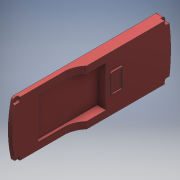
# Autodesk Inventor part: ET10
Saved by Autodesk Inventor 2016 (Build 200138000, 138)
## iProperties
Created: 2016-03-20
Part Number: ET10
Material: Genérico
Document SubType Name: Modeling
Designer: Usuario1
Density: 1 g/cm^3
Appearance: Valor por defecto
Author: Usuario1
Autodesk Inventor part; units mm, degrees
ref_plane "XZ Plane" through (0, 0, 0) normal (0, 1, 0) x (-1, 0, 0)
ref_plane "XY Plane" through (0, 0, 0) normal (0, 0, 1) x (1, 0, 0)
sketch "Boceto1" plane through (0, 0, 0) normal (1, 0, 0) x (0, 1, 0)
  line L0 (5.0799, -0.4268) -> (5.0799, -2.9809)
  line L1 (5.0799, -2.9809) -> (1.2627, -2.9809)
  line L2 (1.2627, -2.9809) -> (1.2627, -0.4268)
  line L3 (1.2627, -0.4268) -> (5.0799, -0.4268)
  line L4 (6.0017, -1.144) -> (6.0017, -2.2637)
  line L5 (6.0017, -2.2637) -> (5.4144, -2.2637)
  line L6 (5.4144, -2.2637) -> (5.4144, -1.144)
  line L7 (5.4144, -1.144) -> (6.0017, -1.144)
  arc A0 (-0.1462, -0.1163) -> (-0.1462, -3.2914) centre (6.7442, -1.7039) ccw
  arc A1 (-0.1462, -3.2914) -> (0, -3.4078) centre (0, -3.2578) ccw
  arc A2 (0, 0) -> (-0.1462, -0.1163) centre (0, -0.15) ccw
  arc A3 (9.0036, -3.2776) -> (9.0036, -0.1302) centre (-2.8031, -1.7039) ccw
  arc A4 (8.8549, -3.4078) -> (9.0036, -3.2776) centre (8.8549, -3.2578) ccw
  arc A5 (9.0036, -0.1302) -> (8.8549, 0) centre (8.8549, -0.15) ccw
  circle A6 centre (8.8549, -0.15) radius 0.092
  line L8 (8.7264, 0) -> (8.7264, -0.16)
  line L9 (9.0226, -0.28) -> (8.8464, -0.28)
  arc A7 (8.7264, -0.16) -> (8.8464, -0.28) centre (8.8464, -0.16) ccw
  circle A8 centre (0, -0.15) radius 0.092
  line L10 (0.1285, 0) -> (0.1285, -0.16)
  line L11 (-0.1818, -0.28) -> (0.0085, -0.28)
  arc A9 (0.0085, -0.28) -> (0.1285, -0.16) centre (0.0085, -0.16) ccw
  circle A10 centre (8.8549, -3.2578) radius 0.092
  line L12 (8.7264, -3.4078) -> (8.7264, -3.2478)
  line L13 (9.0226, -3.1278) -> (8.8464, -3.1278)
  arc A11 (8.8464, -3.1278) -> (8.7264, -3.2478) centre (8.8464, -3.2478) ccw
  circle A12 centre (0, -3.2578) radius 0.092
  line L14 (0.1285, -3.4078) -> (0.1285, -3.2478)
  line L15 (-0.1818, -3.1278) -> (0.0085, -3.1278)
  arc A13 (0.1285, -3.2478) -> (0.0085, -3.1278) centre (0.0085, -3.2478) ccw
  line L16 (8.8549, 0) -> (0, 0)
  line L17 (0, -3.4078) -> (8.8549, -3.4078)
  line L18 (5.8255, -1.144) -> (5.8255, -2.2637)
  line L19 (5.3143, -1.144) -> (5.3143, -2.2637)
  line L20 (5.358, -1.144) -> (5.358, -2.2637)
  line L21 (6.0582, -1.144) -> (6.0582, -2.2637)
  line L22 (6.1019, -1.144) -> (6.1019, -2.2637)
  line L23 (6.0017, -1.0439) -> (5.4144, -1.0439)
  line L24 (6.0017, -1.0876) -> (5.4144, -1.0876)
  line L25 (5.4219, -2.3636) -> (6.0017, -2.3639)
  line L26 (6.0017, -2.3201) -> (5.4144, -2.3201)
  arc A14 (6.0017, -2.3639) -> (6.1019, -2.2637) centre (6.0017, -2.2637) ccw
  arc A15 (6.0017, -2.3201) -> (6.0582, -2.2637) centre (6.0017, -2.2637) ccw
  arc A16 (6.0582, -1.144) -> (6.0017, -1.0876) centre (6.0017, -1.144) ccw
  arc A17 (6.1019, -1.144) -> (6.0017, -1.0439) centre (6.0017, -1.144) ccw
  arc A18 (5.4144, -1.0439) -> (5.3143, -1.144) centre (5.4144, -1.144) ccw
  arc A19 (5.4144, -1.0876) -> (5.358, -1.144) centre (5.4144, -1.144) ccw
  arc A20 (5.358, -2.2637) -> (5.4144, -2.3201) centre (5.4144, -2.2637) ccw
  arc A21 (5.3143, -2.2637) -> (5.4219, -2.3636) centre (5.4144, -2.2637) ccw
  line L27 (1.6627, -0.4268) -> (1.6627, -2.9809)
  line L28 (4.6799, -0.4268) -> (4.6799, -2.9809)
  line L29 (3.8847, -3.4078) -> (3.8847, -2.9809)
  line L30 (3.8847, -0.4268) -> (3.8847, 0)
  line L31 (2.98, -3.4078) -> (2.98, -2.9809)
  line L32 (2.98, -0.4268) -> (2.98, 0)
  line L33 (3.8847, -0.4268) -> (5.0799, -0.4268)
  line L34 (5.0799, -0.4268) -> (5.0799, -2.9809)
  line L35 (5.0799, -2.9809) -> (3.8847, -2.9809)
  constraints: 72 end point, 40 point on circle, 22 centre point, 20 point on line
extrude "Extrusión1" add sketch "Boceto1" along normal blind 0.15 contours L3 L30 L16 L8 A7 L9 A3 L13 A11 L12 L17 L29 L1 L0 | L4 L5 L18 L7 | L18 L5 L6 L7 | A18 L23 A17 L22 A14 L25 A21 L19 | A19 L24 A16 L21 A15 L26 A20 L20
ref_plane "Plano de trabajo1" through (-0.24, 0, 0) normal (1, 0, 0) x (0, 1, 0)
sketch "Boceto2" plane through (-0.24, 0, 0) normal (1, 0, 0) x (0, 1, 0)
  line L0 (5.0799, -0.4268) -> (5.0799, -2.9809)
  line L1 (5.0799, -2.9809) -> (1.2627, -2.9809)
  line L2 (1.2627, -2.9809) -> (1.2627, -0.4268)
  line L3 (1.2627, -0.4268) -> (5.0799, -0.4268)
  line L4 (6.0017, -1.144) -> (6.0017, -2.2637)
  line L5 (6.0017, -2.2637) -> (5.4144, -2.2637)
  line L6 (5.4144, -2.2637) -> (5.4144, -1.144)
  line L7 (5.4144, -1.144) -> (6.0017, -1.144)
  arc A0 (-0.1462, -0.1163) -> (-0.1462, -3.2914) centre (6.7442, -1.7039) ccw
  arc A1 (-0.1462, -3.2914) -> (0, -3.4078) centre (0, -3.2578) ccw
  arc A2 (0, 0) -> (-0.1462, -0.1163) centre (0, -0.15) ccw
  arc A3 (9.0036, -3.2776) -> (9.0036, -0.1302) centre (-2.8031, -1.7039) ccw
  arc A4 (8.8549, -3.4078) -> (9.0036, -3.2776) centre (8.8549, -3.2578) ccw
  arc A5 (9.0036, -0.1302) -> (8.8549, 0) centre (8.8549, -0.15) ccw
  circle A6 centre (8.8549, -0.15) radius 0.092
  line L8 (8.7264, 0) -> (8.7264, -0.16)
  line L9 (9.0226, -0.28) -> (8.8464, -0.28)
  arc A7 (8.7264, -0.16) -> (8.8464, -0.28) centre (8.8464, -0.16) ccw
  circle A8 centre (0, -0.15) radius 0.092
  line L10 (0.1285, 0) -> (0.1285, -0.16)
  line L11 (-0.1818, -0.28) -> (0.0085, -0.28)
  arc A9 (0.0085, -0.28) -> (0.1285, -0.16) centre (0.0085, -0.16) ccw
  circle A10 centre (8.8549, -3.2578) radius 0.092
  line L12 (8.7264, -3.4078) -> (8.7264, -3.2478)
  line L13 (9.0226, -3.1278) -> (8.8464, -3.1278)
  arc A11 (8.8464, -3.1278) -> (8.7264, -3.2478) centre (8.8464, -3.2478) ccw
  circle A12 centre (0, -3.2578) radius 0.092
  line L14 (0.1285, -3.4078) -> (0.1285, -3.2478)
  line L15 (-0.1818, -3.1278) -> (0.0085, -3.1278)
  arc A13 (0.1285, -3.2478) -> (0.0085, -3.1278) centre (0.0085, -3.2478) ccw
  line L16 (8.8549, 0) -> (0, 0)
  line L17 (0, -3.4078) -> (8.8549, -3.4078)
  line L18 (5.8255, -1.144) -> (5.8255, -2.2637)
  line L19 (5.3143, -1.144) -> (5.3143, -2.2637)
  line L20 (5.358, -1.144) -> (5.358, -2.2637)
  line L21 (6.0582, -1.144) -> (6.0582, -2.2637)
  line L22 (6.1019, -1.144) -> (6.1019, -2.2637)
  line L23 (6.0017, -1.0439) -> (5.4144, -1.0439)
  line L24 (6.0017, -1.0876) -> (5.4144, -1.0876)
  line L25 (5.4219, -2.3636) -> (6.0017, -2.3639)
  line L26 (6.0017, -2.3201) -> (5.4144, -2.3201)
  arc A14 (6.0017, -2.3639) -> (6.1019, -2.2637) centre (6.0017, -2.2637) ccw
  arc A15 (6.0017, -2.3201) -> (6.0582, -2.2637) centre (6.0017, -2.2637) ccw
  arc A16 (6.0582, -1.144) -> (6.0017, -1.0876) centre (6.0017, -1.144) ccw
  arc A17 (6.1019, -1.144) -> (6.0017, -1.0439) centre (6.0017, -1.144) ccw
  arc A18 (5.4144, -1.0439) -> (5.3143, -1.144) centre (5.4144, -1.144) ccw
  arc A19 (5.4144, -1.0876) -> (5.358, -1.144) centre (5.4144, -1.144) ccw
  arc A20 (5.358, -2.2637) -> (5.4144, -2.3201) centre (5.4144, -2.2637) ccw
  arc A21 (5.3143, -2.2637) -> (5.4219, -2.3636) centre (5.4144, -2.2637) ccw
  line L27 (1.6627, -0.4268) -> (1.6627, -2.9809)
  line L28 (4.6799, -0.4268) -> (4.6799, -2.9809)
  line L29 (3.8847, -3.4078) -> (3.8847, -2.9809)
  line L30 (3.8847, -0.4268) -> (3.8847, 0)
  line L31 (2.98, -3.4078) -> (2.98, -2.9809)
  line L32 (2.98, -0.4268) -> (2.98, 0)
  line L33 (3.8847, -0.4268) -> (5.0799, -0.4268)
  line L34 (5.0799, -0.4268) -> (5.0799, -2.9809)
  line L35 (5.0799, -2.9809) -> (3.8847, -2.9809)
  line L36 (5.0799, -0.4268) -> (5.0799, -2.9809) projected
  line L37 (3.8847, -0.4268) -> (5.0799, -0.4268) projected
  line L38 (3.8847, 0) -> (3.8847, -0.4268) projected
  line L39 (8.7264, 0) -> (3.8847, 0) projected
  line L40 (8.7264, -0.16) -> (8.7264, 0) projected
  arc A22 (8.7264, -0.16) -> (8.8464, -0.28) centre (8.8464, -0.16) ccw projected
  line L41 (9.0226, -0.28) -> (8.8464, -0.28) projected
  arc A23 (9.0226, -3.1278) -> (9.0226, -0.28) centre (-2.8031, -1.7039) ccw projected
  line L42 (8.8464, -3.1278) -> (9.0226, -3.1278) projected
  arc A24 (8.8464, -3.1278) -> (8.7264, -3.2478) centre (8.8464, -3.2478) ccw projected
  line L43 (8.7264, -3.4078) -> (8.7264, -3.2478) projected
  line L44 (3.8847, -3.4078) -> (8.7264, -3.4078) projected
  line L45 (3.8847, -2.9809) -> (3.8847, -3.4078) projected
  line L46 (5.0799, -2.9809) -> (3.8847, -2.9809) projected
  line L47 (0, -3.4078) -> (2.98, -3.4078)
  line L48 (2.98, 0) -> (0, 0)
  line L49 (2.98, -0.4268) -> (2.98, -2.9809)
  point P0 (0, 0)
  constraints: 78 end point, 40 point on circle, 22 centre point, 20 point on line, 3 collinear
extrude "Extrusión2" add sketch "Boceto2" against normal blind 0.15 contours L49 L1 L27 L3 | L3 L2 L1 L31 L17 L14 A13 L15 A0 L11 A9 L10 L16 L32 | L27 L1 L2 L3 | L17 A1 A0 L15 A13 L14 | A12
sketch "Boceto3" plane through (-0.24, 0.1285, 0) normal (0, 0, 1) x (1, 0, 0)
  line L0 (0.24, 8.5978) -> (0.24, 3.7561) projected
  line L1 (0.24, 3.7561) -> (0.39, 3.7561) projected
  line L2 (0.39, 8.5978) -> (0.39, 3.7561) projected
  line L3 (0.24, 8.5978) -> (0.39, 8.5978) projected
  line L4 (0, 2.8515) -> (0, 0) projected
  line L5 (0, 2.8515) -> (-0.15, 2.8515) projected
  line L6 (-0.15, 0) -> (-0.15, 2.8515) projected
  line L7 (0, 0) -> (-0.15, 0) projected
  arc A0 (0.24, 3.7561) -> (-0.15, 2.8515) centre (1.386, 2.7257) ccw
  line L8 (0.24, 3.7561) -> (0.39, 3.7561) projected
  line L9 (0.24, 3.7561) -> (0.39, 3.7561)
  line L10 (-0.15, 0) -> (-0.15, 2.8515) projected
  line L11 (0, 2.8515) -> (0, 0) projected
  line L12 (-0.15, 2.8515) -> (0, 2.8515)
  arc A1 (0.39, 3.7561) -> (0, 2.8515) centre (1.536, 2.7257) ccw
  line L13 (0.24, 3.7561) -> (0.39, 3.7561)
  line L14 (-0.15, 2.8515) -> (0, 2.8515)
  point P0 (0.24, -0.1285)
  constraints: 8 end point, 6 point on circle, 2 centre point, 2 equal length, 2 horizontal, 2 point on line
extrude "Extrusión3" add sketch "Boceto3" against normal blind 3.4078 contours L1 A1 L5 A0
sketch "Boceto4" plane through (0.15, 0, 0) normal (1, 0, 0) x (0, 0, -1)
  line L0 (0.4268, 5.0799) -> (2.9809, 5.0799) projected
  line L1 (2.9809, 5.0799) -> (2.9809, 3.8847) projected
  line L2 (2.9809, 3.8847) -> (3.4078, 3.8847) projected
  line L3 (3.4078, 3.8847) -> (3.4078, 8.7264) projected
  line L4 (3.4078, 8.7264) -> (3.2478, 8.7264) projected
  arc A0 (3.1278, 8.8464) -> (3.2478, 8.7264) centre (3.2478, 8.8464) ccw projected
  line L5 (3.1278, 8.8464) -> (3.1278, 9.0226) projected
  arc A1 (3.1278, 9.0226) -> (0.28, 9.0226) centre (1.7039, -2.8031) ccw projected
  line L6 (0.28, 9.0226) -> (0.28, 8.8464) projected
  arc A2 (0.16, 8.7264) -> (0.28, 8.8464) centre (0.16, 8.8464) ccw projected
  line L7 (0.16, 8.7264) -> (0, 8.7264) projected
  line L8 (0, 8.7264) -> (0, 3.8847) projected
  line L9 (0, 3.8847) -> (0.4268, 3.8847) projected
  line L10 (0.4268, 3.8847) -> (0.4268, 5.0799) projected
  line L11 (0.4268, 5.0799) -> (2.9809, 5.0799)
  line L12 (2.9809, 5.0799) -> (2.9809, 1.2627)
  line L13 (2.9809, 1.2627) -> (0.4268, 1.2627)
  line L14 (0.4268, 1.2627) -> (0.4268, 5.0799)
  line L15 (1.144, 6.0017) -> (2.2637, 6.0017)
  line L16 (2.2637, 6.0017) -> (2.2637, 5.4144)
  line L17 (2.2637, 5.4144) -> (1.144, 5.4144)
  line L18 (1.144, 5.4144) -> (1.144, 6.0017)
  arc A3 (0.1163, -0.1462) -> (3.2914, -0.1462) centre (1.7039, 6.7442) ccw
  arc A4 (3.2914, -0.1462) -> (3.4078, 0) centre (3.2578, 0) ccw
  arc A5 (0, 0) -> (0.1163, -0.1462) centre (0.15, 0) ccw
  arc A6 (3.2776, 9.0036) -> (0.1302, 9.0036) centre (1.7039, -2.8031) ccw
  arc A7 (3.4078, 8.8549) -> (3.2776, 9.0036) centre (3.2578, 8.8549) ccw
  arc A8 (0.1302, 9.0036) -> (0, 8.8549) centre (0.15, 8.8549) ccw
  circle A9 centre (0.15, 8.8549) radius 0.092
  line L19 (0, 8.7264) -> (0.16, 8.7264)
  line L20 (0.28, 9.0226) -> (0.28, 8.8464)
  arc A10 (0.16, 8.7264) -> (0.28, 8.8464) centre (0.16, 8.8464) ccw
  circle A11 centre (0.15, 0) radius 0.092
  line L21 (0, 0.1285) -> (0.16, 0.1285)
  line L22 (0.28, -0.1818) -> (0.28, 0.0085)
  arc A12 (0.28, 0.0085) -> (0.16, 0.1285) centre (0.16, 0.0085) ccw
  circle A13 centre (3.2578, 8.8549) radius 0.092
  line L23 (3.4078, 8.7264) -> (3.2478, 8.7264)
  line L24 (3.1278, 9.0226) -> (3.1278, 8.8464)
  arc A14 (3.1278, 8.8464) -> (3.2478, 8.7264) centre (3.2478, 8.8464) ccw
  circle A15 centre (3.2578, 0) radius 0.092
  line L25 (3.4078, 0.1285) -> (3.2478, 0.1285)
  line L26 (3.1278, -0.1818) -> (3.1278, 0.0085)
  arc A16 (3.2478, 0.1285) -> (3.1278, 0.0085) centre (3.2478, 0.0085) ccw
  line L27 (0, 8.8549) -> (0, 0)
  line L28 (3.4078, 0) -> (3.4078, 8.8549)
  line L29 (1.144, 5.8255) -> (2.2637, 5.8255)
  line L30 (1.144, 5.3143) -> (2.2637, 5.3143)
  line L31 (1.144, 5.358) -> (2.2637, 5.358)
  line L32 (1.144, 6.0582) -> (2.2637, 6.0582)
  line L33 (1.144, 6.1019) -> (2.2637, 6.1019)
  line L34 (1.0439, 6.0017) -> (1.0439, 5.4144)
  line L35 (1.0876, 6.0017) -> (1.0876, 5.4144)
  line L36 (2.3636, 5.4219) -> (2.3639, 6.0017)
  line L37 (2.3201, 6.0017) -> (2.3201, 5.4144)
  arc A17 (2.3639, 6.0017) -> (2.2637, 6.1019) centre (2.2637, 6.0017) ccw
  arc A18 (2.3201, 6.0017) -> (2.2637, 6.0582) centre (2.2637, 6.0017) ccw
  arc A19 (1.144, 6.0582) -> (1.0876, 6.0017) centre (1.144, 6.0017) ccw
  arc A20 (1.144, 6.1019) -> (1.0439, 6.0017) centre (1.144, 6.0017) ccw
  arc A21 (1.0439, 5.4144) -> (1.144, 5.3143) centre (1.144, 5.4144) ccw
  arc A22 (1.0876, 5.4144) -> (1.144, 5.358) centre (1.144, 5.4144) ccw
  arc A23 (2.2637, 5.358) -> (2.3201, 5.4144) centre (2.2637, 5.4144) ccw
  arc A24 (2.2637, 5.3143) -> (2.3636, 5.4219) centre (2.2637, 5.4144) ccw
  line L38 (0.4268, 1.6627) -> (2.9809, 1.6627)
  line L39 (0.4268, 4.6799) -> (2.9809, 4.6799)
  line L40 (3.4078, 3.8847) -> (2.9809, 3.8847)
  line L41 (0.4268, 3.8847) -> (0, 3.8847)
  line L42 (3.4078, 2.98) -> (2.9809, 2.98)
  line L43 (0.4268, 2.98) -> (0, 2.98)
  line L44 (0.4268, 3.8847) -> (0.4268, 5.0799)
  line L45 (0.4268, 5.0799) -> (2.9809, 5.0799)
  line L46 (2.9809, 5.0799) -> (2.9809, 3.8847)
  point P0 (0, 0)
  constraints: 72 end point, 40 point on circle, 22 centre point, 20 point on line
extrude "Extrusión4" cut sketch "Boceto4" against normal blind 3.4078 contours L39 L1 L12 L38 L14 L10 | L38 L12 L13 L14
ref_plane "Plano de trabajo2" through (-0.52, 0, 0) normal (1, 0, 0) x (0, 1, 0)
sketch "Boceto5" plane through (-0.52, 0, 0) normal (1, 0, 0) x (0, 1, 0)
  arc A0 (9.0226, -3.1278) -> (9.0226, -0.28) centre (-2.8031, -1.7039) ccw projected
  line L0 (5.0799, -0.4268) -> (5.0799, -2.9809)
  line L1 (5.0799, -2.9809) -> (1.2627, -2.9809)
  line L2 (1.2627, -2.9809) -> (1.2627, -0.4268)
  line L3 (1.2627, -0.4268) -> (5.0799, -0.4268)
  line L4 (6.0017, -1.144) -> (6.0017, -2.2637)
  line L5 (6.0017, -2.2637) -> (5.4144, -2.2637)
  line L6 (5.4144, -2.2637) -> (5.4144, -1.144)
  line L7 (5.4144, -1.144) -> (6.0017, -1.144)
  arc A1 (-0.1462, -0.1163) -> (-0.1462, -3.2914) centre (6.7442, -1.7039) ccw
  arc A2 (-0.1462, -3.2914) -> (0, -3.4078) centre (0, -3.2578) ccw
  arc A3 (0, 0) -> (-0.1462, -0.1163) centre (0, -0.15) ccw
  arc A4 (9.0036, -3.2776) -> (9.0036, -0.1302) centre (-2.8031, -1.7039) ccw
  arc A5 (8.8549, -3.4078) -> (9.0036, -3.2776) centre (8.8549, -3.2578) ccw
  arc A6 (9.0036, -0.1302) -> (8.8549, 0) centre (8.8549, -0.15) ccw
  circle A7 centre (8.8549, -0.15) radius 0.092
  line L8 (8.7264, 0) -> (8.7264, -0.16)
  line L9 (9.0226, -0.28) -> (8.8464, -0.28)
  arc A8 (8.7264, -0.16) -> (8.8464, -0.28) centre (8.8464, -0.16) ccw
  circle A9 centre (0, -0.15) radius 0.092
  line L10 (0.1285, 0) -> (0.1285, -0.16)
  line L11 (-0.1818, -0.28) -> (0.0085, -0.28)
  arc A10 (0.0085, -0.28) -> (0.1285, -0.16) centre (0.0085, -0.16) ccw
  circle A11 centre (8.8549, -3.2578) radius 0.092
  line L12 (8.7264, -3.4078) -> (8.7264, -3.2478)
  line L13 (9.0226, -3.1278) -> (8.8464, -3.1278)
  arc A12 (8.8464, -3.1278) -> (8.7264, -3.2478) centre (8.8464, -3.2478) ccw
  circle A13 centre (0, -3.2578) radius 0.092
  line L14 (0.1285, -3.4078) -> (0.1285, -3.2478)
  line L15 (-0.1818, -3.1278) -> (0.0085, -3.1278)
  arc A14 (0.1285, -3.2478) -> (0.0085, -3.1278) centre (0.0085, -3.2478) ccw
  line L16 (8.8549, 0) -> (0, 0)
  line L17 (0, -3.4078) -> (8.8549, -3.4078)
  line L18 (5.8255, -1.144) -> (5.8255, -2.2637)
  line L19 (5.3143, -1.144) -> (5.3143, -2.2637)
  line L20 (5.358, -1.144) -> (5.358, -2.2637)
  line L21 (6.0582, -1.144) -> (6.0582, -2.2637)
  line L22 (6.1019, -1.144) -> (6.1019, -2.2637)
  line L23 (6.0017, -1.0439) -> (5.4144, -1.0439)
  line L24 (6.0017, -1.0876) -> (5.4144, -1.0876)
  line L25 (5.4219, -2.3636) -> (6.0017, -2.3639)
  line L26 (6.0017, -2.3201) -> (5.4144, -2.3201)
  arc A15 (6.0017, -2.3639) -> (6.1019, -2.2637) centre (6.0017, -2.2637) ccw
  arc A16 (6.0017, -2.3201) -> (6.0582, -2.2637) centre (6.0017, -2.2637) ccw
  arc A17 (6.0582, -1.144) -> (6.0017, -1.0876) centre (6.0017, -1.144) ccw
  arc A18 (6.1019, -1.144) -> (6.0017, -1.0439) centre (6.0017, -1.144) ccw
  arc A19 (5.4144, -1.0439) -> (5.3143, -1.144) centre (5.4144, -1.144) ccw
  arc A20 (5.4144, -1.0876) -> (5.358, -1.144) centre (5.4144, -1.144) ccw
  arc A21 (5.358, -2.2637) -> (5.4144, -2.3201) centre (5.4144, -2.2637) ccw
  arc A22 (5.3143, -2.2637) -> (5.4219, -2.3636) centre (5.4144, -2.2637) ccw
  line L27 (1.6627, -0.4268) -> (1.6627, -2.9809)
  line L28 (4.6799, -0.4268) -> (4.6799, -2.9809)
  line L29 (3.8847, -3.4078) -> (3.8847, -2.9809)
  line L30 (3.8847, -0.4268) -> (3.8847, 0)
  line L31 (2.98, -3.4078) -> (2.98, -2.9809)
  line L32 (2.98, -0.4268) -> (2.98, 0)
  line L33 (3.8847, -0.4268) -> (5.0799, -0.4268)
  line L34 (5.0799, -0.4268) -> (5.0799, -2.9809)
  line L35 (5.0799, -2.9809) -> (3.8847, -2.9809)
  arc A23 (0, -0.15) -> (0, -3.2578) centre (6.7442, -1.7039) ccw
  line L36 (0, -3.2578) -> (8.8549, -3.2578)
  arc A24 (8.8549, -3.2578) -> (8.8549, -0.15) centre (-2.8031, -1.7039) ccw
  line L37 (8.8549, -0.15) -> (0, -0.15)
  line L38 (2.98, 0) -> (0.1285, 0) projected
  line L39 (0.1285, 0) -> (8.7264, 0)
  line L40 (8.7264, 0) -> (8.7264, -0.15)
  line L41 (8.7264, -0.15) -> (0.1285, -0.15)
  line L42 (0.1285, -0.15) -> (0.1285, 0)
  line L43 (8.7264, -3.4078) -> (0.1285, -3.4078)
  line L44 (0.1285, -3.4078) -> (0.1285, -3.2578)
  line L45 (0.1285, -3.2578) -> (8.7264, -3.2578)
  line L46 (8.7264, -3.2578) -> (8.7264, -3.4078)
  line L47 (-0.0286, -3.1278) -> (-0.1818, -3.1278)
  arc A25 (-0.1818, -0.28) -> (-0.1462, -3.2914) centre (6.7442, -1.7039) ccw projected
  line L48 (-0.0286, -0.28) -> (-0.1818, -0.28)
  line L49 (9.0226, -0.28) -> (8.8715, -0.28)
  line L50 (9.0226, -0.28) -> (8.8464, -0.28) projected
  line L51 (9.0226, -3.1278) -> (8.8715, -3.1278)
  line L52 (8.8464, -3.1278) -> (9.0226, -3.1278) projected
  arc A26 (0, 0) -> (-0.1462, -0.1163) centre (0, -0.15) ccw
  line L53 (0.0085, -0.28) -> (-0.0286, -0.28)
  line L54 (-0.0286, -0.28) -> (-0.1818, -0.28)
  line L55 (0.1285, -0.16) -> (0.1285, -0.15)
  arc A27 (0.0085, -0.28) -> (0.1285, -0.16) centre (0.0085, -0.16) ccw
  arc A28 (-0.1462, -0.1163) -> (-0.1818, -0.28) centre (6.7442, -1.7039) ccw
  point P0 (0, 0)
  dimension "d10" = 0.15
  constraints: 106 end point, 54 point on circle, 28 point on line, 27 centre point, 4 horizontal, 4 parallel, 3 collinear, 2 perpendicular, 1 concentric, 3 other
  measures "d10" distance between parallel lines of L16 L37
extrude "Extrusión5" add sketch "Boceto5" along normal blind 0.13 contours L13 A24 L9 A0 | A4 A5 L17 L12 L36 A11 A24 L13 | L9 A24 A7 L37 L8 L16 A6 A4 | A24 A11 L36 L12 A12 L13 | L9 A8 L8 L37 A7 A24 | A24 L36 A11 | A11 L36 A24 | A24 L37 A7 | A7 L37 A24 | L17 L29 L36 L12 | L8 L37 L30 L16 | L17 L31 L36 L29 | L30 L37 L32 L16 | L17 L14 L36 L31 | L32 L37 L10 L16 | L17 A2 A1 L15 A23 A13 L36 L14 | L10 L37 A9 A23 L11 A1 A3 L16 | L36 A13 A23 L15 A14 L14 | L10 A10 L11 A23 A9 L37 | L36 A23 A13 | A13 A23 L36 | L37 A23 A9 | A9 A23 L37 | A1 L11 A23 L15
sketch "Boceto6" plane through (-0.39, 0, 0) normal (1, 0, 0) x (0, 0, -1)
  line L0 (0, 2.98) -> (0.15, 2.98) projected
  line L1 (0.15, 2.98) -> (0.15, 8.7264) projected
  line L2 (0.15, 8.7264) -> (0.16, 8.7264) projected
  arc A0 (0.16, 8.7264) -> (0.28, 8.8464) centre (0.16, 8.8464) ccw projected
  line L3 (0.28, 8.8464) -> (0.28, 8.8715) projected
  arc A1 (3.1278, 8.8715) -> (0.28, 8.8715) centre (1.7039, -2.8031) ccw projected
  line L4 (3.1278, 8.8715) -> (3.1278, 8.8464) projected
  arc A2 (3.1278, 8.8464) -> (3.2478, 8.7264) centre (3.2478, 8.8464) ccw projected
  line L5 (3.2478, 8.7264) -> (3.2578, 8.7264) projected
  line L6 (3.2578, 8.7264) -> (3.2578, 2.98) projected
  line L7 (3.2578, 2.98) -> (3.4078, 2.98) projected
  line L8 (3.4078, 2.98) -> (3.4078, 8.7264) projected
  line L9 (3.4078, 8.7264) -> (3.4078, 8.8549) projected
  arc A3 (3.4078, 8.8549) -> (3.2776, 9.0036) centre (3.2578, 8.8549) ccw projected
  arc A4 (3.2776, 9.0036) -> (0.1302, 9.0036) centre (1.7039, -2.8031) ccw projected
  arc A5 (0.1302, 9.0036) -> (0, 8.8549) centre (0.15, 8.8549) ccw projected
  line L10 (0, 8.8549) -> (0, 2.98) projected
  point P0 (0, 0)
extrude "Extrusión6" add sketch "Boceto6" along normal blind 0.15
sketch "Boceto7" plane through (-0.24, 0, 0) normal (1, 0, 0) x (0, 0, -1)
  line L0 (3.4078, 3.5281) -> (3.2578, 3.5281) projected
  line L1 (3.4078, 3.5281) -> (3.4078, 8.7264) projected
  line L2 (3.4078, 8.7264) -> (3.4078, 8.8549) projected
  arc A0 (3.4078, 8.8549) -> (3.2776, 9.0036) centre (3.2578, 8.8549) ccw projected
  arc A1 (3.2776, 9.0036) -> (0.1302, 9.0036) centre (1.7039, -2.8031) ccw projected
  arc A2 (0.1302, 9.0036) -> (0, 8.8549) centre (0.15, 8.8549) ccw projected
  line L3 (0, 8.8549) -> (0, 3.5281) projected
  line L4 (0.15, 3.5281) -> (0, 3.5281) projected
  line L5 (0.15, 3.5281) -> (0.15, 8.7264) projected
  line L6 (0.15, 8.7264) -> (0.16, 8.7264) projected
  arc A3 (0.16, 8.7264) -> (0.28, 8.8464) centre (0.16, 8.8464) ccw projected
  line L7 (0.28, 8.8464) -> (0.28, 8.8715) projected
  arc A4 (3.1278, 8.8715) -> (0.28, 8.8715) centre (1.7039, -2.8031) ccw projected
  line L8 (3.1278, 8.8715) -> (3.1278, 8.8464) projected
  arc A5 (3.1278, 8.8464) -> (3.2478, 8.7264) centre (3.2478, 8.8464) ccw projected
  line L9 (3.2478, 8.7264) -> (3.2578, 8.7264) projected
  line L10 (3.2578, 8.7264) -> (3.2578, 3.5281) projected
  point P0 (0, 0)
extrude "Extrusión7" add sketch "Boceto7" along normal blind 0.15
sketch "Boceto8" plane through (-0.09, 0, 0) normal (1, 0, 0) x (0, 0, -1)
  line L0 (0.15, 3.7748) -> (0, 3.7748) projected
  line L1 (0.15, 3.7748) -> (0.15, 8.7264) projected
  line L2 (0.15, 8.7264) -> (0.16, 8.7264) projected
  arc A0 (0.16, 8.7264) -> (0.28, 8.8464) centre (0.16, 8.8464) ccw projected
  line L3 (0.28, 8.8464) -> (0.28, 8.8715) projected
  arc A1 (3.1278, 8.8715) -> (0.28, 8.8715) centre (1.7039, -2.8031) ccw projected
  line L4 (3.1278, 8.8715) -> (3.1278, 8.8464) projected
  arc A2 (3.1278, 8.8464) -> (3.2478, 8.7264) centre (3.2478, 8.8464) ccw projected
  line L5 (3.2478, 8.7264) -> (3.2578, 8.7264) projected
  line L6 (3.2578, 8.7264) -> (3.2578, 3.7748) projected
  line L7 (3.4078, 3.7748) -> (3.2578, 3.7748) projected
  line L8 (3.4078, 3.7748) -> (3.4078, 8.7264) projected
  line L9 (3.4078, 8.7264) -> (3.4078, 8.8549) projected
  arc A3 (3.4078, 8.8549) -> (3.2776, 9.0036) centre (3.2578, 8.8549) ccw projected
  arc A4 (3.2776, 9.0036) -> (0.1302, 9.0036) centre (1.7039, -2.8031) ccw projected
  arc A5 (0.1302, 9.0036) -> (0, 8.8549) centre (0.15, 8.8549) ccw projected
  line L10 (0, 8.8549) -> (0, 3.7748) projected
  point P0 (0, 0)
extrude "Extrusión8" add sketch "Boceto8" along normal blind 0.15
sketch "Boceto9" plane through (0.15, 5.0799, -0.4268) normal (0, 0, -1) x (-1, 0, 0)
  line L0 (0.15, -1.1953) -> (0.15, 0) projected
  line L1 (0.15, 0) -> (0.15, 0.15)
  line L2 (0.54, -2.0999) -> (0.54, -3.8173) projected
  line L3 (0.54, -3.8173) -> (0.54, -3.9673)
  line L4 (0.54, -3.9673) -> (0.67, -3.9673)
  line L5 (0.67, -4.9514) -> (0.67, 3.6464) projected
  line L6 (0.15, 0.15) -> (0.67, 0.15)
  line L7 (0.67, 0.15) -> (0.67, -3.9673)
  arc A0 (0.54, -2.0999) -> (0.15, -1.1953) centre (-0.996, -2.2257) ccw projected
  point P0 (0.15, -5.0799)
  dimension "d19" = 0.15
  dimension "d20" = 0.15
  dimension "d21" = 0.13
  constraints: 10 end point, 2 point on line, 2 vertical, 1 collinear, 1 horizontal
  measures "d19" distance of L0.end L1.end
  measures "d20" distance of L2.end L3.end
  measures "d21" distance of L3.end L4.end
extrude "Extrusión9" add sketch "Boceto9" against normal blind 0.15
sketch "Boceto10" plane through (0, 5.0799, -2.9809) normal (0, 0, 1) x (1, 0, 0)
  line L0 (0, 0) -> (0.15, 0) projected
  line L1 (0.15, -1.1953) -> (0.15, 0) projected
  arc A0 (0.15, -1.1953) -> (-0.24, -2.0999) centre (1.296, -2.2257) ccw projected
  line L2 (-0.24, -3.8173) -> (-0.24, -2.0999) projected
  line L3 (-0.24, -3.8173) -> (-0.39, -3.8173) projected
  line L4 (-0.39, -3.9673) -> (-0.39, -3.8173) projected
  line L5 (-0.39, -3.9673) -> (-0.52, -3.9673) projected
  line L6 (-0.52, -3.9673) -> (-0.52, 0.15) projected
  line L7 (-0.52, 0.15) -> (0, 0.15) projected
  line L8 (0, 0) -> (0, 0.15) projected
  point P0 (0, -5.0799)
extrude "Extrusión10" add sketch "Boceto10" against normal blind 0.15
sketch "Boceto11" plane through (0.15, 5.0799, -0.4268) normal (0, 0, -1) x (-1, 0, 0)
  line L0 (0.67, 0.15) -> (0.67, -3.9673) projected
  line L1 (0.15, 0.15) -> (0.67, 0.15) projected
  arc A0 (0.54, -2.0999) -> (0.15, -1.1953) centre (-0.996, -2.2257) ccw projected
  line L2 (0.15, 0.15) -> (0.15, -1.1953) projected
  line L3 (0.15, 0.15) -> (0.67, 0.15) projected
  line L4 (0.67, 0.15) -> (0.67, -3.9673) projected
  line L5 (0.67, -3.9673) -> (0.54, -3.9673) projected
  line L6 (0.54, -2.0999) -> (0.54, -3.9673) projected
  line L7 (0.54, -2.0999) -> (0.54, -3.9673) projected
  line L8 (0.54, -3.9673) -> (0.67, -3.9673)
  line L9 (0.67, -3.9673) -> (0.67, 0.15)
  line L10 (0.67, 0.15) -> (0.54, 0.15)
  line L11 (0.54, 0.15) -> (0.54, -3.9673)
  point P0 (0.15, -5.0799)
  constraints: 8 end point, 2 parallel, 1 horizontal, 1 perpendicular
extrude "Extrusión11" add sketch "Boceto11" along normal blind 2.6 contours L0 L5 L6 L11 L1
sketch "Boceto12" plane through (-0.52, 5.2299, -0.2768) normal (0, 1, 0) x (1, 0, 0)
  line L0 (0, 0) -> (0, 2.8541) projected
  line L1 (0.52, 0) -> (0, 0) projected
  line L2 (0.52, 0.15) -> (0.52, 0) projected
  line L3 (0.13, 0.15) -> (0.52, 0.15) projected
  line L4 (0.13, 0.15) -> (0.13, 2.7041) projected
  line L5 (0.13, 2.7041) -> (0.52, 2.7041) projected
  line L6 (0.52, 2.8541) -> (0.52, 2.7041) projected
  line L7 (0, 2.8541) -> (0.52, 2.8541) projected
  line L8 (0.52, 0.15) -> (0.52, 2.7041) projected
  line L9 (0.52, 2.8541) -> (0.52, 2.7041) projected
  line L10 (0.52, 0.15) -> (0.52, 2.7041)
  line L11 (0.52, 0.15) -> (0.13, 0.15)
  line L12 (0.13, 0.15) -> (0.13, 2.7041)
  line L13 (0.13, 2.7041) -> (0.52, 2.7041)
  line L14 (0.52, 2.7041) -> (0.52, 0.15)
  point P0 (0.52, -0.2768)
  constraints: 10 end point, 2 parallel, 1 horizontal, 1 perpendicular, 1 vertical
extrude "Extrusión12" add sketch "Boceto12" against normal blind 0.15 contours L3 L4 L5 L8
sketch "Boceto13" plane through (0.15, 0, 0) normal (1, 0, 0) x (0, 0, -1)
  line L0 (0.4268, 5.0799) -> (2.9809, 5.0799)
  line L1 (2.9809, 5.0799) -> (2.9809, 1.2627)
  line L2 (2.9809, 1.2627) -> (0.4268, 1.2627)
  line L3 (0.4268, 1.2627) -> (0.4268, 5.0799)
  line L4 (1.144, 6.0017) -> (2.2637, 6.0017)
  line L5 (2.2637, 6.0017) -> (2.2637, 5.4144)
  line L6 (2.2637, 5.4144) -> (1.144, 5.4144)
  line L7 (1.144, 5.4144) -> (1.144, 6.0017)
  arc A0 (0.1163, -0.1462) -> (3.2914, -0.1462) centre (1.7039, 6.7442) ccw
  arc A1 (3.2914, -0.1462) -> (3.4078, 0) centre (3.2578, 0) ccw
  arc A2 (0, 0) -> (0.1163, -0.1462) centre (0.15, 0) ccw
  arc A3 (3.2776, 9.0036) -> (0.1302, 9.0036) centre (1.7039, -2.8031) ccw
  arc A4 (3.4078, 8.8549) -> (3.2776, 9.0036) centre (3.2578, 8.8549) ccw
  arc A5 (0.1302, 9.0036) -> (0, 8.8549) centre (0.15, 8.8549) ccw
  circle A6 centre (0.15, 8.8549) radius 0.092
  line L8 (0, 8.7264) -> (0.16, 8.7264)
  line L9 (0.28, 9.0226) -> (0.28, 8.8464)
  arc A7 (0.16, 8.7264) -> (0.28, 8.8464) centre (0.16, 8.8464) ccw
  circle A8 centre (0.15, 0) radius 0.092
  line L10 (0, 0.1285) -> (0.16, 0.1285)
  line L11 (0.28, -0.1818) -> (0.28, 0.0085)
  arc A9 (0.28, 0.0085) -> (0.16, 0.1285) centre (0.16, 0.0085) ccw
  circle A10 centre (3.2578, 8.8549) radius 0.092
  line L12 (3.4078, 8.7264) -> (3.2478, 8.7264)
  line L13 (3.1278, 9.0226) -> (3.1278, 8.8464)
  arc A11 (3.1278, 8.8464) -> (3.2478, 8.7264) centre (3.2478, 8.8464) ccw
  circle A12 centre (3.2578, 0) radius 0.092
  line L14 (3.4078, 0.1285) -> (3.2478, 0.1285)
  line L15 (3.1278, -0.1818) -> (3.1278, 0.0085)
  arc A13 (3.2478, 0.1285) -> (3.1278, 0.0085) centre (3.2478, 0.0085) ccw
  line L16 (0, 8.8549) -> (0, 0)
  line L17 (3.4078, 0) -> (3.4078, 8.8549)
  line L18 (1.144, 5.8255) -> (2.2637, 5.8255)
  line L19 (1.144, 5.3143) -> (2.2637, 5.3143)
  line L20 (1.144, 5.358) -> (2.2637, 5.358)
  line L21 (1.144, 6.0582) -> (2.2637, 6.0582)
  line L22 (1.144, 6.1019) -> (2.2637, 6.1019)
  line L23 (1.0439, 6.0017) -> (1.0439, 5.4144)
  line L24 (1.0876, 6.0017) -> (1.0876, 5.4144)
  line L25 (2.3636, 5.4219) -> (2.3639, 6.0017)
  line L26 (2.3201, 6.0017) -> (2.3201, 5.4144)
  arc A14 (2.3639, 6.0017) -> (2.2637, 6.1019) centre (2.2637, 6.0017) ccw
  arc A15 (2.3201, 6.0017) -> (2.2637, 6.0582) centre (2.2637, 6.0017) ccw
  arc A16 (1.144, 6.0582) -> (1.0876, 6.0017) centre (1.144, 6.0017) ccw
  arc A17 (1.144, 6.1019) -> (1.0439, 6.0017) centre (1.144, 6.0017) ccw
  arc A18 (1.0439, 5.4144) -> (1.144, 5.3143) centre (1.144, 5.4144) ccw
  arc A19 (1.0876, 5.4144) -> (1.144, 5.358) centre (1.144, 5.4144) ccw
  arc A20 (2.2637, 5.358) -> (2.3201, 5.4144) centre (2.2637, 5.4144) ccw
  arc A21 (2.2637, 5.3143) -> (2.3636, 5.4219) centre (2.2637, 5.4144) ccw
  line L27 (0.4268, 1.6627) -> (2.9809, 1.6627)
  line L28 (0.4268, 4.6799) -> (2.9809, 4.6799)
  line L29 (3.4078, 3.8847) -> (2.9809, 3.8847)
  line L30 (0.4268, 3.8847) -> (0, 3.8847)
  line L31 (3.4078, 2.98) -> (2.9809, 2.98)
  line L32 (0.4268, 2.98) -> (0, 2.98)
  line L33 (0.4268, 3.8847) -> (0.4268, 5.0799)
  line L34 (0.4268, 5.0799) -> (2.9809, 5.0799)
  line L35 (2.9809, 5.0799) -> (2.9809, 3.8847)
  arc A22 (3.1278, 9.0226) -> (0.28, 9.0226) centre (1.7039, -2.8031) ccw projected
  point P0 (0, 0)
  constraints: 72 end point, 40 point on circle, 22 centre point, 20 point on line
extrude "Extrusión13" cut sketch "Boceto13" against normal blind 0.26 contours L16 A5 A3 L9 A7 L8 | L12 A11 L13 A3 A4 L17 | A6 | A10
sketch "Boceto14" plane through (0.15, 0, 0) normal (1, 0, 0) x (0, 0, -1)
  line L0 (0.4268, 5.0799) -> (2.9809, 5.0799)
  line L1 (2.9809, 5.0799) -> (2.9809, 1.2627)
  line L2 (2.9809, 1.2627) -> (0.4268, 1.2627)
  line L3 (0.4268, 1.2627) -> (0.4268, 5.0799)
  line L4 (1.144, 6.0017) -> (2.2637, 6.0017)
  line L5 (2.2637, 6.0017) -> (2.2637, 5.4144)
  line L6 (2.2637, 5.4144) -> (1.144, 5.4144)
  line L7 (1.144, 5.4144) -> (1.144, 6.0017)
  arc A0 (0.1163, -0.1462) -> (3.2914, -0.1462) centre (1.7039, 6.7442) ccw
  arc A1 (3.2914, -0.1462) -> (3.4078, 0) centre (3.2578, 0) ccw
  arc A2 (0, 0) -> (0.1163, -0.1462) centre (0.15, 0) ccw
  arc A3 (3.2776, 9.0036) -> (0.1302, 9.0036) centre (1.7039, -2.8031) ccw
  arc A4 (3.4078, 8.8549) -> (3.2776, 9.0036) centre (3.2578, 8.8549) ccw
  arc A5 (0.1302, 9.0036) -> (0, 8.8549) centre (0.15, 8.8549) ccw
  circle A6 centre (0.15, 8.8549) radius 0.092
  line L8 (0, 8.7264) -> (0.16, 8.7264)
  line L9 (0.28, 9.0226) -> (0.28, 8.8464)
  arc A7 (0.16, 8.7264) -> (0.28, 8.8464) centre (0.16, 8.8464) ccw
  circle A8 centre (0.15, 0) radius 0.092
  line L10 (0, 0.1285) -> (0.16, 0.1285)
  line L11 (0.28, -0.1818) -> (0.28, 0.0085)
  arc A9 (0.28, 0.0085) -> (0.16, 0.1285) centre (0.16, 0.0085) ccw
  circle A10 centre (3.2578, 8.8549) radius 0.092
  line L12 (3.4078, 8.7264) -> (3.2478, 8.7264)
  line L13 (3.1278, 9.0226) -> (3.1278, 8.8464)
  arc A11 (3.1278, 8.8464) -> (3.2478, 8.7264) centre (3.2478, 8.8464) ccw
  circle A12 centre (3.2578, 0) radius 0.092
  line L14 (3.4078, 0.1285) -> (3.2478, 0.1285)
  line L15 (3.1278, -0.1818) -> (3.1278, 0.0085)
  arc A13 (3.2478, 0.1285) -> (3.1278, 0.0085) centre (3.2478, 0.0085) ccw
  line L16 (0, 8.8549) -> (0, 0)
  line L17 (3.4078, 0) -> (3.4078, 8.8549)
  line L18 (1.144, 5.8255) -> (2.2637, 5.8255)
  line L19 (1.144, 5.3143) -> (2.2637, 5.3143)
  line L20 (1.144, 5.358) -> (2.2637, 5.358)
  line L21 (1.144, 6.0582) -> (2.2637, 6.0582)
  line L22 (1.144, 6.1019) -> (2.2637, 6.1019)
  line L23 (1.0439, 6.0017) -> (1.0439, 5.4144)
  line L24 (1.0876, 6.0017) -> (1.0876, 5.4144)
  line L25 (2.3636, 5.4219) -> (2.3639, 6.0017)
  line L26 (2.3201, 6.0017) -> (2.3201, 5.4144)
  arc A14 (2.3639, 6.0017) -> (2.2637, 6.1019) centre (2.2637, 6.0017) ccw
  arc A15 (2.3201, 6.0017) -> (2.2637, 6.0582) centre (2.2637, 6.0017) ccw
  arc A16 (1.144, 6.0582) -> (1.0876, 6.0017) centre (1.144, 6.0017) ccw
  arc A17 (1.144, 6.1019) -> (1.0439, 6.0017) centre (1.144, 6.0017) ccw
  arc A18 (1.0439, 5.4144) -> (1.144, 5.3143) centre (1.144, 5.4144) ccw
  arc A19 (1.0876, 5.4144) -> (1.144, 5.358) centre (1.144, 5.4144) ccw
  arc A20 (2.2637, 5.358) -> (2.3201, 5.4144) centre (2.2637, 5.4144) ccw
  arc A21 (2.2637, 5.3143) -> (2.3636, 5.4219) centre (2.2637, 5.4144) ccw
  line L27 (0.4268, 1.6627) -> (2.9809, 1.6627)
  line L28 (0.4268, 4.6799) -> (2.9809, 4.6799)
  line L29 (3.4078, 3.8847) -> (2.9809, 3.8847)
  line L30 (0.4268, 3.8847) -> (0, 3.8847)
  line L31 (3.4078, 2.98) -> (2.9809, 2.98)
  line L32 (0.4268, 2.98) -> (0, 2.98)
  line L33 (0.4268, 3.8847) -> (0.4268, 5.0799)
  line L34 (0.4268, 5.0799) -> (2.9809, 5.0799)
  line L35 (2.9809, 5.0799) -> (2.9809, 3.8847)
  arc A22 (3.1278, 9.0226) -> (0.28, 9.0226) centre (1.7039, -2.8031) ccw projected
  point P0 (0, 0)
  constraints: 72 end point, 40 point on circle, 22 centre point, 20 point on line
extrude "Extrusión14" cut sketch "Boceto14" against normal blind 0.54 contours L10 A9 L11 A0 A2 L16 | L17 A1 A0 L15 A13 L14 | A8 | A12
sketch "Boceto15" plane through (-0.52, 0, 0) normal (-1, 0, 0) x (0, 0, 1)
  line L0 (-3.1309, 5.2299) -> (-0.2768, 5.2299) projected
  line L1 (-0.2768, 5.2299) -> (-0.2768, 3.8847) projected
  line L2 (-0.15, 3.8847) -> (-0.2768, 3.8847) projected
  line L3 (-0.15, 3.8847) -> (-0.15, 8.7264) projected
  line L4 (-0.16, 8.7264) -> (-0.15, 8.7264) projected
  arc A0 (-0.28, 8.8464) -> (-0.16, 8.7264) centre (-0.16, 8.8464) ccw projected
  line L5 (-0.28, 8.8715) -> (-0.28, 8.8464) projected
  arc A1 (-0.28, 8.8715) -> (-3.1278, 8.8715) centre (-1.7039, -2.8031) ccw projected
  line L6 (-3.1278, 8.8464) -> (-3.1278, 8.8715) projected
  arc A2 (-3.2478, 8.7264) -> (-3.1278, 8.8464) centre (-3.2478, 8.8464) ccw projected
  line L7 (-3.2578, 8.7264) -> (-3.2478, 8.7264) projected
  line L8 (-3.2578, 8.7264) -> (-3.2578, 3.8847) projected
  line L9 (-3.1309, 3.8847) -> (-3.2578, 3.8847) projected
  line L10 (-3.1309, 3.8847) -> (-3.1309, 5.2299) projected
  arc A3 (-0.3377, 8.818) -> (-3.07, 8.818) centre (-1.7039, -2.8031) ccw
  arc A4 (-0.3377, 8.818) -> (-0.21, 8.6735) centre (-0.16, 8.8464) ccw
  line L11 (-0.21, 8.6735) -> (-0.21, 3.9447)
  line L12 (-0.21, 3.9447) -> (-0.2168, 3.9447)
  line L13 (-0.2168, 3.9447) -> (-0.2168, 5.2899)
  line L14 (-0.2168, 5.2899) -> (-3.1909, 5.2899)
  line L15 (-3.1909, 5.2899) -> (-3.1909, 3.9447)
  line L16 (-3.1909, 3.9447) -> (-3.1978, 3.9447)
  line L17 (-3.1978, 3.9447) -> (-3.1978, 8.6735)
  arc A5 (-3.1978, 8.6735) -> (-3.07, 8.818) centre (-3.2478, 8.8464) ccw
  line L18 (-3.1978, 8.6735) -> (-3.2578, 8.6735)
  line L19 (-3.07, 8.818) -> (-3.0698, 8.8784)
  arc A6 (-0.28, 8.8715) -> (-3.1278, 8.8715) centre (-1.7039, -2.8031) ccw projected
  arc A7 (-3.0698, 8.8784) -> (-3.1278, 8.8715) centre (-1.7039, -2.8031) ccw
  line L20 (-0.21, 8.6735) -> (-0.15, 8.6735)
  line L21 (-0.15, 0.1285) -> (-0.15, 8.7264) projected
  line L22 (-0.15, 8.7264) -> (-0.15, 8.6735)
  line L23 (-0.3377, 8.818) -> (-0.3377, 8.8784)
  arc A8 (-0.28, 8.8715) -> (-0.3377, 8.8784) centre (-1.7039, -2.8031) ccw
  point P0 (0, 0)
  dimension "d34" = 0.06
  constraints: 24 end point, 13 point on circle, 5 centre point, 3 perpendicular, 2 point on line, 1 parallel, 9 other
  measures "d34" radial gap between concentric circles of A2 A5
extrude "Extrusión15" add sketch "Boceto15" against normal blind 0.54 contours L8 L7 A2 L6 A1 L19 A5 L18 | L20 A4 L23 A1 L5 A0 L4 L3
sketch "Boceto16" plane through (0.15, 0, 0) normal (1, 0, 0) x (0, 0, -1)
  line L0 (2.9809, 3.8847) -> (3.4078, 3.8847) projected
  line L1 (3.4078, 3.8847) -> (3.4078, 8.7264) projected
  line L2 (3.4078, 8.7264) -> (3.2478, 8.7264) projected
  arc A0 (3.1278, 8.8464) -> (3.2478, 8.7264) centre (3.2478, 8.8464) ccw projected
  line L3 (3.1278, 8.8464) -> (3.1278, 9.0226) projected
  arc A1 (3.1278, 9.0226) -> (0.28, 9.0226) centre (1.7039, -2.8031) ccw projected
  line L4 (0.28, 9.0226) -> (0.28, 8.8464) projected
  arc A2 (0.16, 8.7264) -> (0.28, 8.8464) centre (0.16, 8.8464) ccw projected
  line L5 (0.16, 8.7264) -> (0, 8.7264) projected
  line L6 (0, 8.7264) -> (0, 3.8847) projected
  line L7 (0, 3.8847) -> (0.4268, 3.8847) projected
  line L8 (0.4268, 3.8847) -> (0.4268, 5.0799) projected
  line L9 (0.4268, 5.0799) -> (2.9809, 5.0799) projected
  line L10 (2.9809, 5.0799) -> (2.9809, 3.8847) projected
  line L11 (0.4268, 5.0799) -> (2.9809, 5.0799)
  line L12 (2.9809, 5.0799) -> (2.9809, 1.2627)
  line L13 (2.9809, 1.2627) -> (0.4268, 1.2627)
  line L14 (0.4268, 1.2627) -> (0.4268, 5.0799)
  line L15 (1.144, 6.0017) -> (2.2637, 6.0017)
  line L16 (2.2637, 6.0017) -> (2.2637, 5.4144)
  line L17 (2.2637, 5.4144) -> (1.144, 5.4144)
  line L18 (1.144, 5.4144) -> (1.144, 6.0017)
  arc A3 (0.1163, -0.1462) -> (3.2914, -0.1462) centre (1.7039, 6.7442) ccw
  arc A4 (3.2914, -0.1462) -> (3.4078, 0) centre (3.2578, 0) ccw
  arc A5 (0, 0) -> (0.1163, -0.1462) centre (0.15, 0) ccw
  arc A6 (3.2776, 9.0036) -> (0.1302, 9.0036) centre (1.7039, -2.8031) ccw
  arc A7 (3.4078, 8.8549) -> (3.2776, 9.0036) centre (3.2578, 8.8549) ccw
  arc A8 (0.1302, 9.0036) -> (0, 8.8549) centre (0.15, 8.8549) ccw
  circle A9 centre (0.15, 8.8549) radius 0.092
  line L19 (0, 8.7264) -> (0.16, 8.7264)
  line L20 (0.28, 9.0226) -> (0.28, 8.8464)
  arc A10 (0.16, 8.7264) -> (0.28, 8.8464) centre (0.16, 8.8464) ccw
  circle A11 centre (0.15, 0) radius 0.092
  line L21 (0, 0.1285) -> (0.16, 0.1285)
  line L22 (0.28, -0.1818) -> (0.28, 0.0085)
  arc A12 (0.28, 0.0085) -> (0.16, 0.1285) centre (0.16, 0.0085) ccw
  circle A13 centre (3.2578, 8.8549) radius 0.092
  line L23 (3.4078, 8.7264) -> (3.2478, 8.7264)
  line L24 (3.1278, 9.0226) -> (3.1278, 8.8464)
  arc A14 (3.1278, 8.8464) -> (3.2478, 8.7264) centre (3.2478, 8.8464) ccw
  circle A15 centre (3.2578, 0) radius 0.092
  line L25 (3.4078, 0.1285) -> (3.2478, 0.1285)
  line L26 (3.1278, -0.1818) -> (3.1278, 0.0085)
  arc A16 (3.2478, 0.1285) -> (3.1278, 0.0085) centre (3.2478, 0.0085) ccw
  line L27 (0, 8.8549) -> (0, 0)
  line L28 (3.4078, 0) -> (3.4078, 8.8549)
  line L29 (1.144, 5.8255) -> (2.2637, 5.8255)
  line L30 (1.144, 5.3143) -> (2.2637, 5.3143)
  line L31 (1.144, 5.358) -> (2.2637, 5.358)
  line L32 (1.144, 6.0582) -> (2.2637, 6.0582)
  line L33 (1.144, 6.1019) -> (2.2637, 6.1019)
  line L34 (1.0439, 6.0017) -> (1.0439, 5.4144)
  line L35 (1.0876, 6.0017) -> (1.0876, 5.4144)
  line L36 (2.3636, 5.4219) -> (2.3639, 6.0017)
  line L37 (2.3201, 6.0017) -> (2.3201, 5.4144)
  arc A17 (2.3639, 6.0017) -> (2.2637, 6.1019) centre (2.2637, 6.0017) ccw
  arc A18 (2.3201, 6.0017) -> (2.2637, 6.0582) centre (2.2637, 6.0017) ccw
  arc A19 (1.144, 6.0582) -> (1.0876, 6.0017) centre (1.144, 6.0017) ccw
  arc A20 (1.144, 6.1019) -> (1.0439, 6.0017) centre (1.144, 6.0017) ccw
  arc A21 (1.0439, 5.4144) -> (1.144, 5.3143) centre (1.144, 5.4144) ccw
  arc A22 (1.0876, 5.4144) -> (1.144, 5.358) centre (1.144, 5.4144) ccw
  arc A23 (2.2637, 5.358) -> (2.3201, 5.4144) centre (2.2637, 5.4144) ccw
  arc A24 (2.2637, 5.3143) -> (2.3636, 5.4219) centre (2.2637, 5.4144) ccw
  line L38 (0.4268, 1.6627) -> (2.9809, 1.6627)
  line L39 (0.4268, 4.6799) -> (2.9809, 4.6799)
  line L40 (3.4078, 3.8847) -> (2.9809, 3.8847)
  line L41 (0.4268, 3.8847) -> (0, 3.8847)
  line L42 (3.4078, 2.98) -> (2.9809, 2.98)
  line L43 (0.4268, 2.98) -> (0, 2.98)
  line L44 (0.4268, 3.8847) -> (0.4268, 5.0799)
  line L45 (0.4268, 5.0799) -> (2.9809, 5.0799)
  line L46 (2.9809, 5.0799) -> (2.9809, 3.8847)
  point P0 (0, 0)
  constraints: 72 end point, 40 point on circle, 22 centre point, 20 point on line
extrude "Extrusión16" add sketch "Boceto16" along normal blind 0.07 contours A21 L34 A20 L33 A17 L36 A24 L30 | A22 L35 A19 L32 A18 L37 A23 L31
chamfer "Chaflán1" distance 0.069 angle 25 8 edges at (0.22, 5.7081, -1.0439) (0.22, 5.3436, -1.0732) (0.22, 5.3143, -1.7039) (0.22, 5.3463, -2.3371) (0.22, 6.0726, -1.0732) (0.22, 6.1019, -1.7039) (0.22, 6.0726, -2.3345) (0.22, 5.7118, -2.3637) measured on face at (0.22, 5.3443, -1.7039) measured on face at (0.22, 5.7118, -2.3337) measured on face at (0.19, 5.7081, -1.0439) measured on face at (0.22, 5.3667, -2.3152) measured on face at (0.22, 6.0513, -1.0944) measured on face at (0.22, 6.0719, -1.7039) measured on face at (0.22, 6.0513, -2.3133) measured on face at (0.22, 5.3648, -1.0944)
